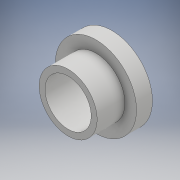
# Autodesk Inventor part: CapForCl
Saved by Autodesk Inventor 2019 (Build 230136000, 136)
## iProperties
Created: 2017-07-24
Part Number: CapForCl
Material: Generic
Document SubType Name: Modeling
Designer: steele
Density: 1 g/cm^3
Appearance: Default
Author: steele
Autodesk Inventor part; units mm, degrees
ref_plane "YZ Plane" through (0, 0, 0) normal (1, 0, 0) x (0, 1, 0)
ref_plane "XZ Plane" through (0, 0, 0) normal (0, 1, 0) x (-1, 0, 0)
ref_plane "XY Plane" through (0, 0, 0) normal (0, 0, 1) x (1, 0, 0)
sketch "Sketch2" plane through (0, 0, 0) normal (0, 0, 1) x (1, 0, 0)
  line L0 (0, 0) -> (0, 9.05) construction
  line L1 (0, 9.05) -> (-8.4, 9.05)
  line L2 (-8.4, 9.05) -> (-8.4, 5.75)
  line L3 (-8.4, 5.75) -> (-6, 5.75)
  line L4 (-6, 5.75) -> (-6, 0)
  line L5 (-6, 0) -> (-4.7743, 0)
  line L6 (0, 0) -> (-6, 0) construction
  line L7 (-4.7743, 0) -> (-4.7743, 6)
  line L8 (0, 9.05) -> (0, 8.5)
  line L9 (-4.7743, 8.5) -> (-4.7743, 6)
  line L10 (-4.7743, 8.5) -> (0, 8.5)
  dimension "d4" = 8.4
  dimension "d5" = 3.3
  dimension "d6" = 5.75
  dimension "d8" = 6
  constraints: 22 end point, 5 perpendicular, 3 vertical, 2 point on line, 1 collinear, 1 horizontal, 1 parallel
  measures "d4" distance of L0.end L1.end
  measures "d5" distance of L1.end L2.end
  measures "d6" distance of L3.end L4.end
  measures "d8" distance between parallel lines of L0 L4
revolve "Revolution1" add sketch "Sketch2" angle 360 about axis through (0, 0, 0) along (0, 1, 0)
sketch "Sketch4" plane through (0, 9.05, 0) normal (0, 1, 0) x (1, 0, 0)
  circle A0 centre (0, 0) radius 8.4 construction
  line L0 (0, -8.4) -> (0, 8.4) construction
  spline S0 degree 2 poles (1.8124, -5.0642) (1.8124, -5.4046) (1.5827, -5.9803) (1.3529, -6.1902) knots 0 0 0 1 2 2 2
  spline S1 degree 2 poles (1.3529, -6.1902) (1.126, -6.4001) (0.4453, -6.6299) (0.0028, -6.6299) knots 0 0 0 1 2 2 2
  spline S2 degree 2 poles (0.0028, -6.6299) (-0.4368, -6.6299) (-1.0891, -6.4058) (-1.3302, -6.1931) knots 0 0 0 1 2 2 2
  spline S3 degree 2 poles (-1.3302, -6.1931) (-1.5656, -5.9832) (-1.8124, -5.4103) (-1.8124, -5.0557) knots 0 0 0 1 2 2 2
  spline S4 degree 2 poles (-1.8124, -5.0557) (-1.8124, -4.8799) (-1.7613, -4.5707) (-1.7216, -4.4402) knots 0 0 0 1 2 2 2
  spline S5 degree 2 poles (-1.7216, -4.4402) (-1.6848, -4.3268) (-1.5798, -4.0914) (-1.5174, -3.9751) knots 0 0 0 1 2 2 2
  line L1 (-1.5174, -3.9751) -> (-0.9558, -3.9751)
  line L2 (-0.9558, -3.9751) -> (-0.9558, -4.012)
  spline S6 degree 2 poles (-0.9558, -4.012) (-1.0126, -4.0744) (-1.1714, -4.2672) (-1.248, -4.4062) knots 0 0 0 1 2 2 2
  spline S7 degree 2 poles (-1.248, -4.4062) (-1.3217, -4.5395) (-1.4153, -4.8543) (-1.4153, -5.0585) knots 0 0 0 1 2 2 2
  spline S8 degree 2 poles (-1.4153, -5.0585) (-1.4153, -5.2826) (-1.231, -5.6825) (-1.0551, -5.8329) knots 0 0 0 1 2 2 2
  spline S9 degree 2 poles (-1.0551, -5.8329) (-0.8764, -5.9803) (-0.3347, -6.1449) (0.0028, -6.1449) knots 0 0 0 1 2 2 2
  spline S10 degree 2 poles (0.0028, -6.1449) (0.363, -6.1449) (0.8821, -5.9718) (1.0608, -5.8215) knots 0 0 0 1 2 2 2
  spline S11 degree 2 poles (1.0608, -5.8215) (1.2338, -5.674) (1.4096, -5.2798) (1.4096, -5.0585) knots 0 0 0 1 2 2 2
  spline S12 degree 2 poles (1.4096, -5.0585) (1.4096, -4.8572) (1.3104, -4.514) (1.2366, -4.3807) knots 0 0 0 1 2 2 2
  spline S13 degree 2 poles (1.2366, -4.3807) (1.1629, -4.253) (1.0097, -4.063) (0.9558, -4.0091) knots 0 0 0 1 2 2 2
  line L3 (0.9558, -4.0091) -> (0.9558, -3.9751)
  line L4 (0.9558, -3.9751) -> (1.5118, -3.9751)
  spline S14 degree 2 poles (1.5118, -3.9751) (1.5656, -4.0914) (1.6649, -4.2956) (1.7103, -4.4402) knots 0 0 0 1 2 2 2
  spline S15 degree 2 poles (1.7103, -4.4402) (1.7613, -4.5934) (1.8124, -4.8543) (1.8124, -5.0642) knots 0 0 0 1 2 2 2
  line L5 (1.75, -3.1242) -> (1.75, -3.5667)
  line L6 (1.75, -3.5667) -> (-1.906, -3.5667)
  line L7 (-1.906, -3.5667) -> (-1.906, -3.1242)
  line L8 (-1.906, -3.1242) -> (1.75, -3.1242)
  spline S16 degree 2 poles (1.8124, 0.4297) (1.8124, 0.0893) (1.5827, -0.4864) (1.3529, -0.6963) knots 0 0 0 1 2 2 2
  spline S17 degree 2 poles (1.3529, -0.6963) (1.126, -0.9062) (0.4453, -1.1359) (0.0028, -1.1359) knots 0 0 0 1 2 2 2
  spline S18 degree 2 poles (0.0028, -1.1359) (-0.4368, -1.1359) (-1.0891, -0.9119) (-1.3302, -0.6991) knots 0 0 0 1 2 2 2
  spline S19 degree 2 poles (-1.3302, -0.6991) (-1.5656, -0.4893) (-1.8124, 0.0837) (-1.8124, 0.4382) knots 0 0 0 1 2 2 2
  spline S20 degree 2 poles (-1.8124, 0.4382) (-1.8124, 0.6141) (-1.7613, 0.9232) (-1.7216, 1.0537) knots 0 0 0 1 2 2 2
  spline S21 degree 2 poles (-1.7216, 1.0537) (-1.6848, 1.1671) (-1.5798, 1.4026) (-1.5174, 1.5188) knots 0 0 0 1 2 2 2
  line L9 (-1.5174, 1.5188) -> (-0.9558, 1.5188)
  line L10 (-0.9558, 1.5188) -> (-0.9558, 1.482)
  spline S22 degree 2 poles (-0.9558, 1.482) (-1.0126, 1.4196) (-1.1714, 1.2267) (-1.248, 1.0877) knots 0 0 0 1 2 2 2
  spline S23 degree 2 poles (-1.248, 1.0877) (-1.3217, 0.9544) (-1.4153, 0.6396) (-1.4153, 0.4354) knots 0 0 0 1 2 2 2
  spline S24 degree 2 poles (-1.4153, 0.4354) (-1.4153, 0.2113) (-1.231, -0.1886) (-1.0551, -0.3389) knots 0 0 0 1 2 2 2
  spline S25 degree 2 poles (-1.0551, -0.3389) (-0.8764, -0.4864) (-0.3347, -0.6509) (0.0028, -0.6509) knots 0 0 0 1 2 2 2
  spline S26 degree 2 poles (0.0028, -0.6509) (0.363, -0.6509) (0.8821, -0.4779) (1.0608, -0.3276) knots 0 0 0 1 2 2 2
  spline S27 degree 2 poles (1.0608, -0.3276) (1.2338, -0.1801) (1.4096, 0.2141) (1.4096, 0.4354) knots 0 0 0 1 2 2 2
  spline S28 degree 2 poles (1.4096, 0.4354) (1.4096, 0.6368) (1.3104, 0.9799) (1.2366, 1.1132) knots 0 0 0 1 2 2 2
  spline S29 degree 2 poles (1.2366, 1.1132) (1.1629, 1.2409) (1.0097, 1.4309) (0.9558, 1.4848) knots 0 0 0 1 2 2 2
  line L11 (0.9558, 1.4848) -> (0.9558, 1.5188)
  line L12 (0.9558, 1.5188) -> (1.5118, 1.5188)
  spline S30 degree 2 poles (1.5118, 1.5188) (1.5656, 1.4026) (1.6649, 1.1983) (1.7103, 1.0537) knots 0 0 0 1 2 2 2
  spline S31 degree 2 poles (1.7103, 1.0537) (1.7613, 0.9005) (1.8124, 0.6396) (1.8124, 0.4297) knots 0 0 0 1 2 2 2
  spline S32 degree 2 poles (1.472, 3.3823) (1.5118, 3.3284) (1.6536, 3.1469) (1.6961, 3.0618) knots 0 0 0 1 2 2 2
  spline S33 degree 2 poles (1.6961, 3.0618) (1.7585, 2.9455) (1.8237, 2.7271) (1.8237, 2.5286) knots 0 0 0 1 2 2 2
  spline S34 degree 2 poles (1.8237, 2.5286) (1.8237, 2.3669) (1.7018, 2.0748) (1.5912, 1.9641) knots 0 0 0 1 2 2 2
  spline S35 degree 2 poles (1.5912, 1.9641) (1.4834, 1.8592) (1.1657, 1.7316) (0.9899, 1.7316) knots 0 0 0 1 2 2 2
  spline S36 degree 2 poles (0.9899, 1.7316) (0.7176, 1.7316) (0.3318, 1.9613) (0.2212, 2.2109) knots 0 0 0 1 2 2 2
  spline S37 degree 2 poles (0.2212, 2.2109) (0.1191, 2.4321) (0.0425, 3.0334) (0.0227, 3.3823) knots 0 0 0 1 2 2 2
  line L13 (0.0227, 3.3823) -> (-0.0624, 3.3823)
  spline S38 degree 2 poles (-0.0624, 3.3823) (-0.2156, 3.3823) (-0.4056, 3.2887) (-0.4595, 3.2036) knots 0 0 0 1 2 2 2
  spline S39 degree 2 poles (-0.4595, 3.2036) (-0.5134, 3.1185) (-0.5474, 2.8746) (-0.5474, 2.7441) knots 0 0 0 1 2 2 2
  spline S40 degree 2 poles (-0.5474, 2.7441) (-0.5474, 2.591) (-0.4566, 2.1769) (-0.3687, 1.9698) knots 0 0 0 1 2 2 2
  line L14 (-0.3687, 1.9698) -> (-0.3687, 1.9443)
  line L15 (-0.3687, 1.9443) -> (-0.8197, 1.9443)
  spline S41 degree 2 poles (-0.8197, 1.9443) (-0.8537, 2.0662) (-0.9388, 2.5229) (-0.9388, 2.747) knots 0 0 0 1 2 2 2
  spline S42 degree 2 poles (-0.9388, 2.747) (-0.9388, 3.0192) (-0.8537, 3.3908) (-0.7431, 3.5383) knots 0 0 0 1 2 2 2
  spline S43 degree 2 poles (-0.7431, 3.5383) (-0.6353, 3.6829) (-0.2921, 3.8248) (-0.0454, 3.8248) knots 0 0 0 1 2 2 2
  line L16 (-0.0454, 3.8248) -> (1.75, 3.8248)
  line L17 (1.75, 3.8248) -> (1.75, 3.3823)
  line L18 (1.75, 3.3823) -> (1.472, 3.3823)
  line L19 (1.1033, 3.3823) -> (0.3744, 3.3823)
  spline S44 degree 2 poles (0.3744, 3.3823) (0.3886, 3.2235) (0.4368, 2.7441) (0.4822, 2.5938) knots 0 0 0 1 2 2 2
  spline S45 degree 2 poles (0.4822, 2.5938) (0.5361, 2.4179) (0.7601, 2.1882) (0.9587, 2.1882) knots 0 0 0 1 2 2 2
  spline S46 degree 2 poles (0.9587, 2.1882) (1.1856, 2.1882) (1.4153, 2.4435) (1.4153, 2.6874) knots 0 0 0 1 2 2 2
  spline S47 degree 2 poles (1.4153, 2.6874) (1.4153, 2.8944) (1.2366, 3.2348) (1.1033, 3.3823) knots 0 0 0 1 2 2 2
  spline S48 degree 2 poles (0.3659, 6.6469) (1.0239, 6.6469) (1.8011, 6.0201) (1.8011, 5.5407) knots 0 0 0 1 2 2 2
  spline S49 degree 2 poles (1.8011, 5.5407) (1.8011, 5.345) (1.7103, 5.0444) (1.6167, 4.8884) knots 0 0 0 1 2 2 2
  line L20 (1.6167, 4.8884) -> (2.7172, 4.8884)
  line L21 (2.7172, 4.8884) -> (2.7172, 4.4459)
  line L22 (2.7172, 4.4459) -> (-0.8764, 4.4459)
  line L23 (-0.8764, 4.4459) -> (-0.8764, 4.8884)
  line L24 (-0.8764, 4.8884) -> (-0.6013, 4.8884)
  spline S50 degree 2 poles (-0.6013, 4.8884) (-0.7516, 5.0529) (-0.9502, 5.4556) (-0.9502, 5.691) knots 0 0 0 1 2 2 2
  spline S51 degree 2 poles (-0.9502, 5.691) (-0.9502, 6.142) (-0.2354, 6.6469) (0.3659, 6.6469) knots 0 0 0 1 2 2 2
  spline S52 degree 2 poles (0.4169, 6.1902) (-0.034, 6.1902) (-0.5304, 5.9038) (-0.5304, 5.5833) knots 0 0 0 1 2 2 2
  spline S53 degree 2 poles (-0.5304, 5.5833) (-0.5304, 5.3961) (-0.363, 5.0444) (-0.2326, 4.8884) knots 0 0 0 1 2 2 2
  line L25 (-0.2326, 4.8884) -> (1.2593, 4.8884)
  spline S54 degree 2 poles (1.2593, 4.8884) (1.3416, 5.0614) (1.404, 5.3081) (1.404, 5.467) knots 0 0 0 1 2 2 2
  spline S55 degree 2 poles (1.404, 5.467) (1.404, 5.8102) (0.8991, 6.1902) (0.4169, 6.1902) knots 0 0 0 1 2 2 2
  constraints: 2 end point, 2 point on circle, 2 vertical
extrude "Extrusion1" cut sketch "Sketch4" against normal blind 0.5
body "Solid1"
